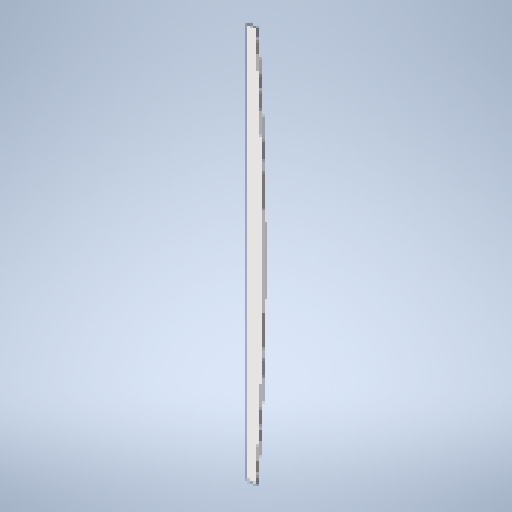
# Autodesk Inventor part: MSC 0512 rib back mould
Saved by Autodesk Inventor 2025 (Build 290162010, 162A)
## iProperties
Created: 2024-04-18
Part Number: MSC 0512 rib back mould
Material: AISI304
Document SubType Name: Sheet Metal
Designer: admin
Stock Number: МОО 024 лист борт основной
Mass: 48027.3 g
Surface Area: 40202.8 cm^2
Volume: 6003.41 cm^3
Density: 8 g/cm^3
Sheet Metal Rule: Default
Sheet Metal Width: 72,741 mm
Sheet Metal Length: 1700,000 mm
Sheet Metal Area: 123659,382 mm^2
Appearance: Default
Flat Pattern Width: 7.27408 cm
Flat Pattern Length: 170 cm
Flat Pattern Area: 1236.59 cm^2
Author: admin
Autodesk Inventor part; units mm, degrees
ref_plane "YZ Plane" through (0, 0, 0) normal (1, 0, 0) x (0, 1, 0)
ref_plane "XZ Plane" through (0, 0, 0) normal (0, 1, 0) x (-1, 0, 0)
ref_plane "XY Plane" through (0, 0, 0) normal (0, 0, 1) x (1, 0, 0)
sketch "Sketch1" plane through (0, 0, 0) normal (0, 0, 1) x (1, 0, 0)
  arc A0 (40, -850) -> (40, 850) centre (-10977.2592, 0) ccw
  line L0 (0, -850) -> (40, -850)
  line L1 (40, 850) -> (0, 850)
  line L2 (0, 850) -> (0, -850)
  point P0 (0, 0)
  point P1 (0, 0)
  dimension "d121" = 1700
  dimension "d122" = 40
  dimension "d128" = 11050
  measures "d121" distance of L1.end L0.start
  measures "d122" distance of L0.end L0.start
  measures "d128" radius of A0
extrude "Plate3" add sketch "Sketch1" along normal blind 2
body "Solid4"
